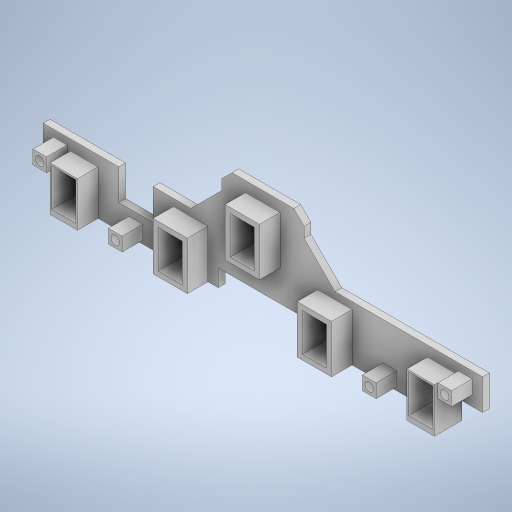
# Autodesk Inventor part: Infravermelhos_revisto_2
Saved by Autodesk Inventor 2024 (Build 280153000, 153)
## iProperties
Created: 2023-04-03
Part Number: Infravermelhos_revisto_2
Material: Generic
Document SubType Name: Modeling
Designer: guilh
Density: 1 g/cm^3
Appearance: Default
Author: guilh
Autodesk Inventor part; units mm, degrees
ref_plane "YZ Plane" through (0, 0, 0) normal (1, 0, 0) x (0, 1, 0)
ref_plane "XZ Plane" through (0, 0, 0) normal (0, 1, 0) x (-1, 0, 0)
ref_plane "XY Plane" through (0, 0, 0) normal (0, 0, 1) x (1, 0, 0)
sketch "Sketch1" plane through (0, 0, 0) normal (0, 0, 1) x (1, 0, 0)
  line L0 (-64, 31) -> (-73, 31)
  line L1 (-76, 28) -> (-76, 25)
  line L2 (-85, 16) -> (-76, 25)
  line L3 (-76, 28) -> (-73, 31)
  line L4 (-64, 31) -> (-55, 31)
  line L5 (-52, 28) -> (-52, 25)
  line L6 (-43, 16) -> (-52, 25)
  line L7 (-52, 28) -> (-55, 31)
  line L8 (-43, 16) -> (0, 16)
  line L9 (-77, 0) -> (-77, 5)
  line L10 (-77, 5) -> (-51, 5)
  line L11 (-51, 5) -> (-51, 0)
  line L12 (-106, 16) -> (-106, 7)
  line L13 (-106, 7) -> (-96, 7)
  line L14 (-96, 7) -> (-96, 16)
  line L15 (-128, 16) -> (-106, 16)
  line L16 (-96, 16) -> (-85, 16)
  line L17 (-120, 0) -> (-120, 7)
  line L18 (-120, 7) -> (-128, 7)
  line L19 (-120, 0) -> (-77, 0)
  line L20 (-128, 16) -> (-128, 7)
  line L21 (-8, 0) -> (-8, 7)
  line L22 (-8, 7) -> (0, 7)
  line L23 (-51, 0) -> (-8, 0)
  line L24 (0, 7) -> (0, 16)
  point P0 (0, 0)
  dimension "d0" = 128
  dimension "d6" = 3
  dimension "d67" = 5
  dimension "d71" = 22
  dimension "d74" = 9
  dimension "d75" = 10
  dimension "d93" = 7
  dimension "d94" = 8
  dimension "d95" = 7
  constraints: 50 end point, 6 horizontal, 3 perpendicular, 2 vertical
  measures "d0" distance of L15.start L8.end
  measures "d6" distance of L1.start L1.end
  measures "d67" distance of L9.start L9.end
  measures "d71" distance of L15.start L12.start
  measures "d74" distance of L12.start L12.end
  measures "d75" distance of L12.end L13.end
  measures "d93" distance of L17.start L17.end
  measures "d94" distance of point (0, 0) L21.start
  measures "d95" distance of L21.start L21.end
extrude "Extrusion1" add sketch "Sketch1" against normal blind 2
sketch "Sketch2" plane through (0, 0, 0) normal (0, 0, 1) x (1, 0, 0)
  line L0 (-121, 10) -> (-125, 10)
  line L1 (-125, 10) -> (-125, 14)
  line L2 (-125, 14) -> (-121, 14)
  line L3 (-121, 14) -> (-121, 10)
  line L4 (-90, 0) -> (-80, 0)
  line L5 (-80, 0) -> (-80, 14)
  line L6 (-80, 14) -> (-90, 14)
  line L7 (-90, 14) -> (-90, 0)
  line L8 (-99, 1) -> (-103, 1)
  line L9 (-103, 1) -> (-103, 5)
  line L10 (-103, 5) -> (-99, 5)
  line L11 (-99, 5) -> (-99, 1)
  line L12 (-7, 10) -> (-3, 10)
  line L13 (-3, 10) -> (-3, 14)
  line L14 (-3, 14) -> (-7, 14)
  line L15 (-7, 14) -> (-7, 10)
  line L16 (-29, 1) -> (-25, 1)
  line L17 (-25, 1) -> (-25, 5)
  line L18 (-25, 5) -> (-29, 5)
  line L19 (-29, 5) -> (-29, 1)
  line L20 (-112, 13) -> (-120, 13)
  line L21 (-120, 13) -> (-120, 0)
  line L22 (-112, 13) -> (-112, 0)
  circle A0 centre (-123, 12) radius 1.25
  circle A1 centre (-101, 3) radius 1.25
  circle A2 centre (-27, 3) radius 1.25
  circle A3 centre (-5, 12) radius 1.25
  line L23 (-120, 0) -> (-112, 0)
  line L24 (-119.5, 12.5) -> (-119.5, 1.5)
  line L25 (-119.5, 1.5) -> (-112.5, 1.5)
  line L26 (-112.5, 1.5) -> (-112.5, 12.5)
  line L27 (-112.5, 12.5) -> (-119.5, 12.5)
  line L28 (-88.5, 12.5) -> (-88.5, 1.5)
  line L29 (-88.5, 1.5) -> (-81.5, 1.5)
  line L30 (-81.5, 1.5) -> (-81.5, 12.5)
  line L31 (-81.5, 12.5) -> (-88.5, 12.5)
  line L32 (-69, 14) -> (-59, 14)
  line L33 (-59, 14) -> (-59, 28)
  line L34 (-59, 28) -> (-69, 28)
  line L35 (-69, 28) -> (-69, 14)
  line L36 (-67.5, 26.5) -> (-67.5, 15.5)
  line L37 (-67.5, 15.5) -> (-60.5, 15.5)
  line L38 (-60.5, 15.5) -> (-60.5, 26.5)
  line L39 (-60.5, 26.5) -> (-67.5, 26.5)
  line L40 (-38, 0) -> (-48, 0)
  line L41 (-48, 0) -> (-48, 14)
  line L42 (-48, 14) -> (-38, 14)
  line L43 (-38, 14) -> (-38, 0)
  line L44 (-16, 13) -> (-8, 13)
  line L45 (-8, 13) -> (-8, 0)
  line L46 (-16, 13) -> (-16, 0)
  line L47 (-8, 0) -> (-16, 0)
  line L48 (-8.5, 12.5) -> (-8.5, 1.5)
  line L49 (-8.5, 1.5) -> (-15.5, 1.5)
  line L50 (-15.5, 1.5) -> (-15.5, 12.5)
  line L51 (-15.5, 12.5) -> (-8.5, 12.5)
  line L52 (-39.5, 12.5) -> (-39.5, 1.5)
  line L53 (-39.5, 1.5) -> (-46.5, 1.5)
  line L54 (-46.5, 1.5) -> (-46.5, 12.5)
  line L55 (-46.5, 12.5) -> (-39.5, 12.5)
  dimension "d49" = 2.5
  dimension "d50" = 2.5
  dimension "d51" = 2.5
  dimension "d52" = 2.5
  dimension "d69" = 13
  constraints: 112 end point, 12 perpendicular, 8 parallel, 4 centre point, 3 vertical, 2 horizontal
  measures "d49" diameter of A0
  measures "d50" diameter of A1
  measures "d51" diameter of A2
  measures "d52" diameter of A3
  measures "d69" distance of L22.end L20.start
sketch "Sketch10" plane through (0, 0, 0) normal (0, 0, 1) x (1, 0, 0)
  line L0 (-121, 10) -> (-125, 10)
  line L1 (-125, 10) -> (-125, 14)
  line L2 (-125, 14) -> (-121, 14)
  line L3 (-121, 14) -> (-121, 10)
  line L4 (-25, 1) -> (-25, 5)
  line L5 (-7, 14) -> (-7, 10)
  line L6 (-7, 10) -> (-3, 10)
  line L7 (-3, 10) -> (-3, 14)
  line L8 (-3, 14) -> (-7, 14)
  line L9 (-29, 1) -> (-25, 1)
  line L10 (-25, 5) -> (-29, 5)
  line L11 (-29, 5) -> (-29, 1)
  circle A0 centre (-123, 12) radius 1.25
  circle A1 centre (-27, 3) radius 1.25
  circle A2 centre (-5, 12) radius 1.25
  line L12 (-90, 0) -> (-80, 0)
  line L13 (-80, 0) -> (-80, 14)
  line L14 (-80, 14) -> (-90, 14)
  line L15 (-90, 14) -> (-90, 0)
  line L16 (-99, 1) -> (-103, 1)
  line L17 (-103, 1) -> (-103, 5)
  line L18 (-103, 5) -> (-99, 5)
  line L19 (-99, 5) -> (-99, 1)
  line L20 (-112, 13) -> (-120, 13)
  line L21 (-120, 13) -> (-120, 0)
  line L22 (-112, 13) -> (-112, 0)
  circle A3 centre (-101, 3) radius 1.25
  line L23 (-120, 0) -> (-112, 0)
  line L24 (-119.5, 12.5) -> (-119.5, 1.5)
  line L25 (-119.5, 1.5) -> (-112.5, 1.5)
  line L26 (-112.5, 1.5) -> (-112.5, 12.5)
  line L27 (-112.5, 12.5) -> (-119.5, 12.5)
  line L28 (-88.5, 12.5) -> (-88.5, 1.5)
  line L29 (-88.5, 1.5) -> (-81.5, 1.5)
  line L30 (-81.5, 1.5) -> (-81.5, 12.5)
  line L31 (-81.5, 12.5) -> (-88.5, 12.5)
  line L32 (-69, 14) -> (-59, 14)
  line L33 (-59, 14) -> (-59, 28)
  line L34 (-59, 28) -> (-69, 28)
  line L35 (-69, 28) -> (-69, 14)
  line L36 (-67.5, 26.5) -> (-67.5, 15.5)
  line L37 (-60.5, 26.5) -> (-67.5, 26.5)
  line L38 (-60.5, 15.5) -> (-60.5, 26.5)
  line L39 (-67.5, 15.5) -> (-60.5, 15.5)
  line L40 (-15.5, 1.5) -> (-15.5, 12.5)
  line L41 (-16, 13) -> (-16, 0)
  line L42 (-8.5, 1.5) -> (-15.5, 1.5)
  line L43 (-8, 0) -> (-16, 0)
  line L44 (-8.5, 12.5) -> (-8.5, 1.5)
  line L45 (-8, 13) -> (-8, 0)
  line L46 (-15.5, 12.5) -> (-8.5, 12.5)
  line L47 (-16, 13) -> (-8, 13)
  line L48 (-38, 0) -> (-48, 0)
  line L49 (-48, 0) -> (-48, 14)
  line L50 (-48, 14) -> (-38, 14)
  line L51 (-38, 14) -> (-38, 0)
  line L52 (-39.5, 12.5) -> (-39.5, 1.5)
  line L53 (-39.5, 1.5) -> (-46.5, 1.5)
  line L54 (-46.5, 1.5) -> (-46.5, 12.5)
  line L55 (-46.5, 12.5) -> (-39.5, 12.5)
  point P0 (-100.5385, 17.107)
  point P1 (-110.5385, 3.107)
  point P2 (-100.5385, 3.107)
  point P3 (-141.5385, 3.107)
  point P4 (-131.5385, 3.107)
  point P5 (-183.5385, 3.107)
  point P6 (-173.5385, 3.107)
  point P7 (-214.5385, 3.107)
  point P8 (-204.5385, 3.107)
  point P9 (-214.5385, 17.107)
  point P10 (0, 16)
  point P11 (0, 0)
  dimension "d62" = 2.5
  dimension "d64" = 2.5
  dimension "d65" = 2.5
  constraints: 112 end point, 12 perpendicular, 8 parallel, 4 centre point, 3 vertical, 2 horizontal
  measures "d62" diameter of A0
  measures "d64" diameter of A1
  measures "d65" diameter of A2
extrude "Extrusion2" cut sketch "Sketch2" against normal blind 2 contours A0 | A1 | A2 | A3 | L27 L26 L25 L24 | L31 L30 L29 L28 | L39 L38 L37 L36 | L48 L49 L50 L51 | L52 L53 L54 L55
extrude "Extrusion7" add sketch "Sketch10" along normal blind 6
body "Solid1"
